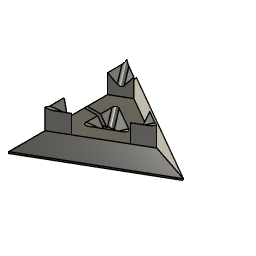
LEDCube Stand (Autodesk Fusion 360 design; units mm, degrees)
Autodesk Fusion 360 part; units mm, degrees
sketch "Sketch4" plane through (0, 0, 0) normal (0, 0, 1) x (1, 0, 0)
  line L0 (0, 0) -> (100, 0)
  line L1 (100, 0) -> (100, 100)
  line L2 (100, 100) -> (0, 100)
  line L3 (0, 100) -> (0, 0)
  dimension "d14" = 100
  dimension "d15" = 100
  constraint horizontal L0
  constraint vertical L1
  constraint horizontal L2
  constraint vertical L3
  constraint coincident L0.start L3.end
  measures "d14" distance of L0.start L0.end
  measures "d15" distance of L0.start L2.end
extrude "Extrude4" add sketch "Sketch4" along normal blind 100 makes body 1
move_body "Move11" bodies 1 to x (1, 0, 0) y (0, 0.707107, 0.707107) z (0, -0.707107, 0.707107) at (0, 0, 0)
move_body "Move12" bodies 1 to x (0.819152, 0, 0.573576) y (0, 1, 0) z (-0.573576, 0, 0.819152) at (0, 0, 0)
fillet "Fillet2" radius 2.5 12 edges at (-60.837, 35.3553, 86.8842) (21.0782, -35.3553, 144.2418) (-60.837, -35.3553, 86.8842) (21.0782, 35.3553, 144.2418) (40.9576, 0, 28.6788) (61.6362, 35.3553, 86.319) (0.3996, 70.7107, 86.6016) (-20.279, 35.3553, 28.9614) (-40.1584, 0, 144.5244) (-20.279, -35.3553, 28.9614) (0.3996, -70.7107, 86.6016) (61.6362, -35.3553, 86.319) 6 faces at (13.7857, -23.5702, 38.4268) (-40.2916, -23.5702, 115.6572) (-40.2916, 23.5702, 115.6572) (0.2664, 47.1405, 57.7344) (-40.558, 23.5702, 57.9228) (27.8379, 0, 134.588) on bodies 1
sketch "Sketch5" plane through (0, 0, 0) normal (0, 0, 1) x (1, 0, 0)
  line L0 (-25, -43.3013) -> (50, 0)
  line L1 (50, 0) -> (-25, 43.3013)
  line L2 (-25, 43.3013) -> (-25, -43.3013)
  dimension "d21" = 25
  constraint vertical L2
  measures "d21" distance of origin L2
extrude "Extrude5" add sketch "Sketch5" along normal blind 10 separate body makes body 2
sketch "Sketch6" plane through (0, 0, 0) normal (0, 0, 1) x (1, 0, 0)
  circle A0 centre (0, 0) radius 3
  line L0 (-25, -1) -> (-2.8284, -1)
  line L1 (-2.8284, -1) -> (-2.8284, 1)
  line L2 (-2.8284, 1) -> (-25, 1)
  line L3 (-25, 1) -> (-25, -1)
  line L4 (-25, 43.3013) -> (-25, -43.3013)
  line L5 (-25, -2.5) -> (-1.6583, -2.5)
  line L6 (-1.6583, -2.5) -> (-1.6583, 2.5)
  line L7 (-1.6583, 2.5) -> (-25, 2.5)
  line L8 (-25, 2.5) -> (-25, -2.5)
  dimension "d24" = 6
  dimension "d28" = 2
  dimension "d39" = 5
  constraint coincident A0.centre origin
  constraint horizontal L0
  constraint vertical L1
  constraint horizontal L2
  constraint vertical L3
  constraint coincident A0 L1.end
  constraint coincident L0.start L4
  constraint coincident A0 L0.end
  constraint horizontal L5
  constraint vertical L6
  constraint horizontal L7
  constraint vertical L8
  constraint coincident A0 L6.end
  constraint coincident L4 L5.start
  constraint coincident A0 L5.end
  measures "d24" diameter of A0
  measures "d28" distance of L0.end L1.end
  measures "d39" distance of L5.end L6.end
extrude "Extrude6" cut sketch "Sketch6" along normal up to surface (10 mm away) contours A0 L6 | A0 L1 L6 | A0 L1 bodies 2
chamfer "Chamfer2" distance 9 angle 45 3 edges at (-25, 0, 10) (12.5, -21.6506, 10) (12.5, 21.6506, 10) on bodies 2
sketch "Sketch7" plane through (0, 0, 10) normal (0, 0, 1) x (-1, 0, 0)
  circle A0 centre (0, 0) radius 3
  line L0 (16, 27.7128) -> (-32, 0)
  line L1 (-32, 0) -> (16, -27.7128)
  line L2 (16, -27.7128) -> (16, 27.7128)
  line L3 (16, 27.7128) -> (0, 0) construction
  line L4 (16, 14.7128) -> (4.7417, 21.2128)
  dimension "d32" = 13
  constraint coincident L0.start L2.end
  constraint coincident A0.centre L3.end
  constraint coincident L2 L4.start
  constraint coincident L0 L4.end
  constraint perpendicular L3 L4
  measures "d32" distance of L4.start L4.end
extrude "Extrude8" add sketch "Sketch7" along normal blind 16 contours L0 L2 L4 bodies 2
pattern_circular "C-Pattern1" count 3 over 360 about axis through (0, 0, 1.75) along (0, 0, 1) of "Extrude8"
combine "Combine2" operation cut target body 2 tool bodies 1 keep tools
extrude "Extrude9" cut sketch "Sketch6" along normal up to surface (10 mm away) contours A0 L0 L2 L3 L4 L8 bodies 2
extrude "Extrude10" cut sketch "Sketch6" along normal blind 4 contours A0 L2 L4 L7 L8 | A0 L0 L4 L5 L8 bodies 2
hidden bodies 1
named bodies: "Cube", "Stand"
